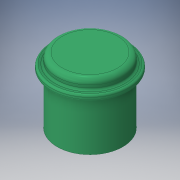
# Autodesk Inventor part: Quiz Part B
Saved by Autodesk Inventor 2016 (Build 200138000, 138)
## iProperties
Created: 2017-01-27
Part Number: Quiz Part B
Material: Generic
Document SubType Name: Modeling
Designer: Dave
Density: 1 g/cm^3
Appearance: Smooth - Dark Sea Green
Author: Dave
Autodesk Inventor part; units mm, degrees
ref_plane "YZ Plane" through (0, 0, 0) normal (1, 0, 0) x (0, 1, 0)
ref_plane "XZ Plane" through (0, 0, 0) normal (0, 1, 0) x (-1, 0, 0)
ref_plane "XY Plane" through (0, 0, 0) normal (0, 0, 1) x (1, 0, 0)
sketch "Sketch1" plane through (0, 0, 0) normal (1, 0, 0) x (0, 1, 0)
  line L0 (0, 0) -> (25.4, 0)
  line L1 (25.4, 0) -> (25.4, -12.7)
  line L2 (25.4, -12.7) -> (0, -12.7)
  line L3 (0, -12.7) -> (0, 0)
  dimension "d1" = 12.7
  dimension "d2" = 25.4
  constraints: 8 end point, 2 perpendicular, 1 horizontal
  measures "d1" distance between parallel lines of L2 L0
  measures "d2" distance between parallel lines of L1 L3
revolve "Revolution1" add sketch "Sketch1" angle 360 about axis through (0, 0, 0) along (0, 1, 0)
fillet "Fillet1" radius 2.032 1 edges at (0, 25.4, 12.7)
shell "Shell1" thickness 1.27 removed faces 1 at (0.9542, 0, 3.6254)
sketch "Sketch4" plane through (0, 0, 0) normal (1, 0, 0) x (0, 1, 0)
  line L0 (24.13, 10.668) -> (24.13, -10.668) projected
  arc A0 (23.368, -11.43) -> (24.13, -10.668) centre (23.368, -10.668) ccw projected
  line L1 (23.368, -11.43) -> (0, -11.43) projected
  line L2 (24.13, -6.35) -> (4.7625, -6.35)
  line L3 (4.7625, -6.35) -> (4.7625, -11.43)
  line L4 (21.1657, 0) -> (0, 0) construction
  line L5 (0, 12.7) -> (0, -12.7) projected
  dimension "d37" = 6.35
  dimension "d38" = 4.7625
  constraints: 6 end point, 2 horizontal, 2 point on line, 1 perpendicular
  measures "d37" distance between parallel lines of L2 L4
  measures "d38" distance between parallel lines of L3 L5
extrude "Extrusion3" add sketch "Sketch4" along normal mid plane 1.524
fillet "Fillet8" radius 1.016 1 edges at (0, 4.7625, -6.35)
sketch "Sketch5" plane through (0, 0, 0) normal (1, 0, 0) x (0, 1, 0)
  line L0 (4.7625, -11.4046) -> (4.7625, -7.366) projected
  line L1 (5.7785, -6.35) -> (24.13, -6.35) projected
  line L2 (7.0576, -6.35) -> (7.9375, -4.826)
  line L3 (7.9375, -4.826) -> (8.8174, -6.35)
  point P0 (0, 0)
  point P1 (18.7869, -3.2512)
  point P2 (24.13, -6.35)
  dimension "d42" = 1.524
  dimension "d43" = 60
  dimension "d44" = 3.175
  constraints: 4 end point, 1 equal length, 3 other
  measures "d43" angle of L3 L2
  measures "d44" distance from line of L2.end L0
extrude "Extrusion4" add sketch "Sketch5" along normal mid plane 1.524
pattern_linear "Rectangular Pattern2" count 4 spacing 2.032 along (0, 1, 0) of "Extrusion4"
pattern_circular "Circular Pattern2" count 4 over 360 about axis through (0, -10, 0) along (0, 1, 0) of "Extrusion3", "Fillet8", "Extrusion4", "Rectangular Pattern2"
sketch "Sketch7" plane through (0, 0, 0) normal (1, 0, 0) x (0, 1, 0)
  line L0 (19.304, -12.7) -> (21.59, -12.7)
  line L1 (21.59, -12.7) -> (21.59, -14.986)
  line L2 (21.59, -14.986) -> (19.304, -14.986)
  line L3 (19.304, -14.986) -> (19.304, -12.7)
  line L4 (23.368, -12.7) -> (0, -12.7) projected
  line L5 (0, 12.7) -> (0, -12.7) projected
  line L6 (-3.4036, 0) -> (20.4216, 0) projected
  point P0 (0, 0)
  dimension "d58" = 21.59
  dimension "d59" = 2.286
  constraints: 8 end point, 2 parallel, 2 perpendicular, 1 horizontal, 1 point on line
  measures "d58" distance between parallel lines of L1 L5
  measures "d59" distance of L1.end L2.end
revolve "Revolution3" add sketch "Sketch7" angle 360 about axis through (0, -10, 0) along (0, 1, 0)
fillet "Fillet10" radius 0.762 4 edges at (0, 21.59, 14.986) (0, 19.304, 14.986) (0, 21.59, 12.7) (0, 19.304, 12.7)
body "Solid1"
